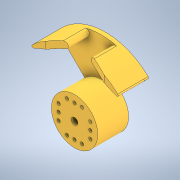
# Autodesk Inventor part: pizza_disk
Saved by Autodesk Inventor 2020 (Build 240168000, 168)
## iProperties
Created: 2022-07-27
Part Number: pizza_disk
Material: Типовые
Document SubType Name: Modeling
Designer: akapu
Density: 1 g/cm^3
Appearance: По умолчанию
Author: akapu
Autodesk Inventor part; units mm, degrees
ref_plane "YZ Plane" through (0, 0, 0) normal (1, 0, 0) x (0, 1, 0)
ref_plane "XZ Plane" through (0, 0, 0) normal (0, 1, 0) x (-1, 0, 0)
ref_plane "XY Plane" through (0, 0, 0) normal (0, 0, 1) x (1, 0, 0)
sketch "Эскиз1" plane through (0, 0, 0) normal (0, 0, 1) x (1, 0, 0)
  circle A0 centre (0, 0) radius 30
  circle A1 centre (0, 0) radius 25
  circle A2 centre (0, 0) radius 28
  line L0 (0, 0) -> (28, 0) construction
  line L1 (0, 0) -> (28, 0) construction
  line L2 (0, 28) -> (-5.2, 28)
  line L3 (-5.2, 28) -> (-5.2, 24.4532)
  line L4 (0, 0) -> (19.799, 19.799)
  line L5 (0, 0) -> (28, 0) construction
  line L6 (-0.4901, 1.1812) -> (26.3238, 1.1812) construction
  line L7 (0, 0) -> (-19.799, 19.799)
  line L8 (0, 0) -> (28, 0) construction
  line L9 (-5.2, 24.4532) -> (5.2, 24.4532)
  line L10 (5.2, 24.4532) -> (5.2, 28)
  line L11 (5.2, 28) -> (0, 28)
  point P0 (4.9999, 24.4949)
  point P1 (-19.4504, 20.1415)
  point P2 (-5.2, 27.5129)
  dimension "d0" = 60
  dimension "d1" = 50
  dimension "d2" = 56
  dimension "d5" = 5.2
  dimension "d7" = 45
  dimension "d11" = 135
  dimension "d19" = 10.4
  constraints: 24 end point, 7 point on circle, 6 horizontal, 3 centre point, 3 coincident, 2 equal length, 2 perpendicular, 2 tangent
  measures "d0" diameter of A0
  measures "d1" diameter of A1
  measures "d2" diameter of A2
  measures "d5" distance of L2.start L2.end
  measures "d7" angle of L5 L4
  measures "d11" angle of L8 L7
  measures "d19" distance of L3.end L9.end
extrude "Выдавливание1" add sketch "Эскиз1" along normal blind 2 contours L9 A1 | L10 A2 L4 A1 | A1 L4 L7 L9 | A1 L3 A2 L10 | A1 L7 A2 L3
sketch "Эскиз2" plane through (0, 0, 2) normal (0, 0, 1) x (1, 0, 0)
  line L0 (-19.799, 19.799) -> (0, 0) projected
  circle A0 centre (0, 0) radius 25
  line L1 (-5.2, 28) -> (-5.2, 27.5129) projected
  circle A1 centre (0, 0) radius 28
  arc A2 (19.799, 19.799) -> (-19.799, 19.799) centre (0, 0) ccw projected
  line L2 (-5.2, 27.5129) -> (-5.2, 24.4532)
  line L3 (0, 0) -> (19.799, 19.799) projected
  line L4 (19.799, 19.799) -> (17.6777, 17.6777)
  line L5 (-19.799, 19.799) -> (-17.6777, 17.6777)
  line L6 (-5.2, 24.4532) -> (5.2, 24.4532)
  line L7 (5.2, 24.4532) -> (5.2, 27.5129)
  point P0 (4.9999, 24.4949)
  point P1 (4.9874, 27.5522)
  point P2 (0, 28)
  dimension "d20" = 10.4
  constraints: 10 end point, 7 point on circle, 2 centre point, 2 coincident, 2 point on line, 1 collinear, 1 perpendicular, 1 vertical
  measures "d20" distance of L2.end L6.end
extrude "Выдавливание2" add sketch "Эскиз2" along normal blind 11.8 contours A1 L2 A0 L0 | A1 L3 A0 L7
fillet "Сопряжение1" radius 1.5 4 edges at (5.2, 27.5129, 7.9) (5.2, 24.4532, 7.9) (-5.2, 27.5129, 7.9) (-5.2, 24.4532, 7.9)
sketch "Эскиз4" plane through (0, 0, 2) normal (0, 0, 1) x (1, 0, 0)
  line L0 (-17.6777, 17.6777) -> (0, 0) projected
  circle A0 centre (0, 0) radius 10.5
  dimension "d25" = 21
  constraints: 1 centre point, 1 coincident
  measures "d25" diameter of A0
extrude "Выдавливание3" add sketch "Эскиз4" along normal blind 12 and the other way blind 2
sketch "Эскиз3" plane through (0, 0, 2) normal (0, 0, 1) x (1, 0, 0)
  line L0 (0, 28) -> (0, 29)
  line L1 (0, 29) -> (-5, 29)
  line L2 (-5, 29) -> (-5, 19)
  line L3 (-5, 19) -> (5, 19)
  line L4 (0, 29) -> (5, 29)
  line L5 (5, 29) -> (5, 19)
  line L6 (-1.7678, 18.2322) -> (-10, 10)
  line L7 (-19.799, 19.799) -> (-7.4246, 7.4246) projected
  line L8 (1.7678, 18.2322) -> (10, 10)
  line L9 (7.4246, 7.4246) -> (17.6777, 17.6777) projected
  line L10 (10, 10) -> (7.8787, 7.8787)
  circle A0 centre (0, 0) radius 11.1421
  line L11 (-10, 10) -> (-7.8787, 7.8787)
  arc A1 (1.7678, 18.2322) -> (-1.7678, 18.2322) centre (0, 16.4645) ccw
  line L12 (-10, 10) -> (-2.9289, 17.0711)
  line L13 (-2.9289, 17.0711) -> (-10, 24.1421)
  line L14 (-10, 24.1421) -> (-17.0711, 17.0711)
  line L15 (-10, 10) -> (-17.0711, 17.0711)
  line L16 (-7.4246, 7.4246) -> (0, 0)
  arc A2 (7.4246, 7.4246) -> (-7.4246, 7.4246) centre (0, 0) ccw projected
  line L17 (0, 0) -> (7.4246, 7.4246)
  circle A3 centre (0, 0) radius 28
  circle A4 centre (0, 0) radius 25
  line L18 (0, 11.1421) -> (0, 35.3553)
  line L19 (10, 10) -> (27.088, -7.088)
  line L20 (-10, 10) -> (-27.088, -7.088)
  line L21 (27.088, -7.088) -> (-27.088, -7.088)
  line L22 (-17.0711, 17.0711) -> (-21.6622, 12.4799)
  line L23 (-21.6622, 12.4799) -> (-27.1, 7.0422)
  line L24 (10, 10) -> (17.0711, 17.0711)
  line L25 (17.0711, 17.0711) -> (21.6622, 12.4799)
  line L26 (21.6622, 12.4799) -> (12.4799, 21.6622)
  arc A5 (17.6777, 17.6777) -> (6.3208, 24.1878) centre (0, 0) ccw projected
  dimension "d21" = 1
  dimension "d22" = 5
  dimension "d23" = 10
  dimension "d24" = 10
  dimension "d31" = 3
  dimension "d32" = 2.5
  dimension "d33" = 10
  dimension "d34" = 10
  dimension "d35" = 22.2843
  dimension "d36" = 16.4645
  dimension "d37" = 7.8223
  dimension "d38" = 10
  constraints: 50 end point, 12 point on circle, 12 point on line, 9 perpendicular, 4 centre point, 3 coincident, 2 collinear, 2 tangent, 2 vertical, 1 horizontal
  measures "d21" distance of L0.start L0.end
  measures "d22" distance of L0.end L1.end
  measures "d23" distance of L1.end L2.end
  measures "d24" distance of L2.end L3.end
  measures "d31" distance of L8.end L10.end
  measures "d32" radius of A1
  measures "d33" distance of L6.end L12.end
  measures "d34" distance of L12.end L13.end
  measures "d35" diameter of A0
  measures "d36" distance of A1.centre A0.centre
  measures "d38" distance of L8.end L24.end
sketch "Эскиз5" plane through (0, 0, 13.8) normal (0, 0, 1) x (1, 0, 0)
  line L0 (-19.799, 19.799) -> (-7.4246, 7.4246) projected
  line L1 (-19.799, 19.799) -> (-19.0919, 19.0919)
  line L2 (-19.0919, 19.0919) -> (-9.6913, 23.0452)
  arc A0 (-6.3208, 24.1878) -> (-17.6777, 17.6777) centre (0, 0) ccw projected
  line L3 (17.6777, 17.6777) -> (19.799, 19.799) projected
  line L4 (19.799, 19.799) -> (19.0919, 19.0919)
  line L5 (19.0919, 19.0919) -> (9.6913, 23.0452)
  arc A1 (17.6777, 17.6777) -> (6.3208, 24.1878) centre (0, 0) ccw projected
  line L6 (7.4246, 7.4246) -> (17.6777, 17.6777) projected
  line L7 (19.0919, 19.0919) -> (17.6777, 17.6777)
  line L8 (-19.0919, 19.0919) -> (-17.6777, 17.6777)
  circle A2 centre (0, 0) radius 25
  dimension "d39" = 1
  dimension "d40" = 1
  constraints: 12 end point, 2 collinear, 2 point on circle, 1 coincident, 1 point on line, 1 tangent, 3 other
  measures "d39" distance of L0.start L1.end
  measures "d40" distance of L3.end L4.end
extrude "Выдавливание4" cut sketch "Эскиз5" against normal blind 11.8 contours L2 A0 L0 | A1 L5 L3
fillet "Сопряжение2" radius 0.595 4 edges at (19.799, 19.799, 6.9) (19.0919, 19.0919, 7.9) (-19.799, 19.799, 6.9) (-19.0919, 19.0919, 7.9)
sketch "Эскиз6" plane through (0, 0, 14) normal (0, 0, 1) x (1, 0, 0)
  circle A0 centre (0, 0) radius 1.5
  dimension "d44" = 3
  constraints: 1 centre point, 1 coincident
  measures "d44" diameter of A0
extrude "Выдавливание5" cut sketch "Эскиз6" against normal blind 14
sketch "Эскиз7" plane through (0, 0, 14) normal (0, 0, 1) x (1, 0, 0)
  circle A0 centre (0, 0) radius 1.5 projected
  line L0 (0, 0) -> (-7.2, 0)
  circle A1 centre (-7.2, 0) radius 0.75
  line L1 (-7.2, 0) -> (-7.2, 3.4)
  line L2 (-7.2, 3.4) -> (-7.2, -3.4)
  circle A2 centre (-7.2, 3.4) radius 0.75
  circle A3 centre (-7.2, -3.4) radius 0.75
  dimension "d47" = 7.2
  dimension "d48" = 1.5
  dimension "d49" = 3.4
  dimension "d50" = 6.8
  dimension "d51" = 1.5
  dimension "d52" = 1.5
  constraints: 6 end point, 3 centre point, 3 coincident, 1 horizontal, 1 point on line, 1 vertical
  measures "d47" distance of L0.start L0.end
  measures "d48" diameter of A1
  measures "d49" distance of L1.start L1.end
  measures "d50" distance of L1.end L2.end
  measures "d51" diameter of A2
  measures "d52" diameter of A3
extrude "Выдавливание6" cut sketch "Эскиз7" against normal blind 14 contours A3 | A2 | A1 L2 L0 | L0 L1 A1 | L2 A1 L1
pattern_circular "Круговой массив1" count 4 over 360 about axis through (0, 0, 14) along (0, 0, -1) of "Выдавливание6"
sketch "Эскиз8" plane through (0, 0, 0) normal (0, 0, -1) x (-1, 0, 0)
  circle A0 centre (0, 0) radius 1.5 projected
  circle A1 centre (0, 0) radius 1.5 projected
  circle A2 centre (0, 0) radius 9
  dimension "d61" = 18
  constraints: 1 centre point, 1 coincident
  measures "d61" diameter of A2
extrude "Выдавливание7" cut sketch "Эскиз8" against normal blind 4
sketch "Эскиз12" plane through (0, 0, 13.8) normal (0, 0, 1) x (1, 0, 0)
  arc A0 (-7.0792, 27.0903) -> (-19.3619, 20.2267) centre (0, 0) ccw projected
  arc A1 (7.0792, 27.0903) -> (6.3208, 24.1878) centre (6.7, 25.639) ccw projected
  line L0 (-7.0792, 27.0903) -> (7.0792, 27.0903)
  line L1 (7.0792, 27.0903) -> (7.0792, 24.1878)
  line L2 (7.0792, 24.1878) -> (-7.0792, 24.1878)
  line L3 (-7.0792, 24.1878) -> (-7.0792, 27.0903)
  constraints: 8 end point, 3 perpendicular, 1 horizontal
extrude "Выдавливание8" add sketch "Эскиз12" along normal blind 11.8 contours L1 L2 A1 L0 | A1 L2 L3 L0
sketch "Эскиз13" plane through (-6.3208, 27.0903, 13.8) normal (0, 1, 0) x (1, 0, 0)
  line L0 (11.5208, 11.8) -> (11.5208, 0) projected
  line L1 (11.5208, 0) -> (11.5208, 2.2)
  line L2 (11.5208, 2.2) -> (19.5413, 0)
  line L3 (13.4, 0) -> (25.6826, 0) projected
  line L4 (11.5208, 0) -> (19.5413, 0)
  line L5 (12.6415, 0) -> (0, 0) projected
  line L6 (1.1208, 11.8) -> (1.1208, 0) projected
  line L7 (1.1208, 0) -> (1.1208, 2.2)
  line L8 (1.1208, 2.2) -> (-6.8998, 0)
  line L9 (-13.0411, 0) -> (-0.7585, 0) projected
  line L10 (1.1208, 0) -> (0, 0) projected
  line L11 (1.1208, 0) -> (-6.8998, 0)
  line L12 (-0.7585, 11.8) -> (-0.7585, 0) projected
  line L13 (13.4, -11.8) -> (-0.7585, -11.8) projected
  line L14 (-0.7585, 0) -> (-0.7585, -11.8)
  line L15 (-0.7585, -11.8) -> (13.4, -11.8)
  line L16 (13.4, 0) -> (13.4, -11.8) projected
  line L17 (13.4, -11.8) -> (13.4, 0)
  line L18 (13.4, 0) -> (-0.7585, 0)
  point P0 (6.3208, 13.8)
  dimension "d64" = 2.2
  constraints: 20 end point, 5 point on line, 3 collinear, 2 midpoint, 2 perpendicular, 1 vertical
  measures "d64" distance of L1.start L1.end
extrude "Выдавливание9" cut sketch "Эскиз13" against normal mid plane 11.8
sketch "Эскиз15" plane through (0, 0, 4) normal (0, 0, -1) x (-1, 0, 0)
  circle A0 centre (0, 0) radius 2.1
  circle A1 centre (0, 0) radius 1.5 projected
  dimension "d67" = 4.2
  constraints: 1 centre point, 1 coincident
  measures "d67" diameter of A0
extrude "Выдавливание10" add sketch "Эскиз15" along normal blind 0.2
